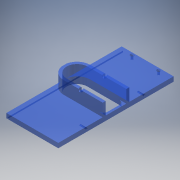
# Autodesk Inventor part: Wand1
Saved by Autodesk Inventor 2018 (Build 220112000, 112)
## iProperties
Created: 2013-02-21
Part Number: Wand1
Material: Polycarbonate, Smoke
Document SubType Name: Modeling
Designer: Neef
Mass: 105.37 g
Surface Area: 310.912 cm^2
Volume: 87.8083 cm^3
Density: 1.2 g/cm^3
Appearance: Clear - Blue
Author: Neef
Autodesk Inventor part; units mm, degrees
ref_plane "YZ Plane" through (0, 0, 0) normal (1, 0, 0) x (0, 1, 0)
ref_plane "XZ Plane" through (0, 0, 0) normal (0, 1, 0) x (-1, 0, 0)
ref_plane "XY Plane" through (0, 0, 0) normal (0, 0, 1) x (1, 0, 0)
sketch "Skizze1" plane through (0, 0, 0) normal (0, 0, 1) x (1, 0, 0)
  line L0 (45, 100) -> (-45, 100)
  line L1 (-45, 100) -> (-45, -100)
  line L2 (-45, -100) -> (45, -100)
  line L3 (45, -100) -> (45, 100)
  line L4 (0, 140) -> (0, -140) projected
  line L5 (-63, 0) -> (63, 0) projected
  point P0 (0, 0)
  point P1 (45, 0)
  point P2 (0, -100)
  dimension "d0" = 200
  dimension "d1" = 90
  constraints: 8 end point, 2 midpoint, 2 parallel, 2 point on line, 1 horizontal, 1 perpendicular
  measures "d0" distance of L2.end L0.start
  measures "d1" distance of L0.start L0.end
extrude "Extrusion1" add sketch "Skizze1" along normal blind 8
sketch "Skizze2" plane through (0, 0, 8) normal (0, 0, 1) x (1, 0, 0)
  line L0 (45, 100) -> (45, -100) projected
  line L1 (-45, -100) -> (-45, 100) projected
  line L2 (45, -18) -> (-22.5, -18)
  arc A0 (-40.5, 0) -> (-22.5, -18) centre (-22.5, 0) ccw
  line L3 (-40.5, 0) -> (-45, 0)
  arc A1 (-45, -4.7697) -> (-22.5, -23) centre (-22.5, 0) ccw
  line L4 (-22.5, -23) -> (45, -23)
  line L5 (0, 140) -> (0, -140) projected
  line L6 (-66.8751, 0) -> (63.6458, 0) projected
  line L7 (-45, -4.7697) -> (-45, 0)
  point P0 (0, 0)
  dimension "d4" = 5
  dimension "d5" = 67.5
  dimension "d6" = 18
  constraints: 8 end point, 5 point on line, 4 point on circle, 2 centre point, 2 perpendicular, 2 tangent, 1 collinear, 1 midpoint, 1 parallel
  measures "d4" distance between parallel lines of L2 L4
  measures "d5" distance of L2.start L2.end
  measures "d6" distance between parallel lines of L6 L2
extrude "Extrusion2" add sketch "Skizze2" along normal blind 22 contours L0 L4 L5 L2 | L5 L4 A1 L1 L3 A0 L2
mirror "Spiegeln1" about plane through (-45, 0, 8) normal (0, 1, 0) of "Extrusion2"
sketch "Skizze3" plane through (0, 0, 8) normal (0, 0, 1) x (1, 0, 0)
  line L0 (45, 18) -> (-22.5, 18) projected
  arc A0 (-22.5, 18) -> (-22.5, -18) centre (-22.5, 0) ccw projected
  line L1 (-22.5, -18) -> (45, -18) projected
  line L2 (45, 18) -> (45, -18) projected
  arc A1 (23, -18) -> (23, 18) centre (23, 0) ccw
  line L3 (-63, 0) -> (63, 0) projected
  line L4 (-22.5, 18) -> (45, 18) projected
  line L5 (-22.5, -18) -> (45, -18) projected
  point P0 (0, 0)
  dimension "d9" = 22
  constraints: 3 point on line, 2 point on circle, 2 tangent, 1 centre point
  measures "d9" distance from line of L2 A1.centre
extrude "Extrusion3" cut sketch "Skizze3" against normal through all contours A1 L3 A0 L0 | A1 L1 A0 L3
sketch "Skizze4" plane through (-45, 100, 0) normal (0, 1, 0) x (1, 0, 0)
  line L0 (90, 0) -> (0, 0) projected
  line L1 (0, 0) -> (0, -8) projected
  line L2 (22.5, -30) -> (22.5, -30) projected
  line L3 (22.5, -30) -> (22.5, 0) projected
  line L4 (22.5, 0) -> (22.5, 0) projected
  line L5 (22.5, 0) -> (22.5, -30) projected
  line L6 (4.5, -30) -> (4.5, 0) projected
  line L7 (2, 0) -> (3.2, 0)
  line L8 (3.2, 0) -> (3.2, -2.5)
  line L9 (3.2, -2.5) -> (2, -2.5)
  line L10 (2, -2.5) -> (2, 0)
  point P0 (45, 0)
  dimension "d12" = 1.2
  dimension "d13" = 2.5
  dimension "d14" = 2
  constraints: 8 end point, 2 parallel, 1 horizontal, 1 perpendicular, 1 point on line
  measures "d12" distance of L8.end L9.end
  measures "d13" distance of L9.end L7.start
  measures "d14" distance between parallel lines of L1 L10
extrude "Extrusion4" cut sketch "Skizze4" against normal through all
sketch "Skizze5" plane through (0, 0, 8) normal (0, 0, 1) x (1, 0, 0)
  arc A0 (23, -18) -> (23, 18) centre (23, 0) ccw projected
  line L0 (45, 18) -> (23, 18) projected
  line L1 (41, 0) -> (41, 10)
  line L2 (33, 18) -> (23, 18)
  arc A1 (41, 0) -> (23, 18) centre (23, 0) ccw
  arc A2 (41, 10) -> (33, 18) centre (33, 10) ccw
  point P0 (0, 0)
  point P1 (41, 18)
  dimension "d17" = 8
  constraints: 5 point on circle, 4 end point, 4 tangent, 3 point on line, 2 centre point, 1 coincident, 1 collinear, 1 perpendicular
  measures "d17" radius of A2
extrude "Extrusion5" cut sketch "Skizze5" against normal up to surface (8 mm away)
mirror "Spiegeln2" about plane through (0, 0, 0) normal (0, 1, 0) of "Extrusion5"
sketch "Skizze6" plane through (45, -100, 0) normal (1, 0, 0) x (0, 0, -1)
  line L0 (-8, 77) -> (-8, 0) projected
  line L1 (0, 0) -> (-8, 0) projected
  point P0 (0, 100)
  point P1 (-4, 50)
  dimension "d20" = 4
  dimension "d21" = 50
  measures "d20" distance from line of L0 point (-4, 50)
  measures "d21" distance from line of point (-4, 50) L1
hole "Bohrung1" at (45, -50, 4) direction (-1, 0, 0) diameter 2.459 depth 12 tip angle 118 thread size "M3x0.5" class "6H" standard "ISO Metric profile"
mirror "Spiegeln3" about plane through (0, 0, 0) normal (0, 1, 0) of "Bohrung1"
sketch "Skizze7" plane through (0, 0, 30) normal (0, 0, 1) x (1, 0, 0)
  line L0 (45, -18) -> (45, -23) projected
  line L1 (-22.5, 18) -> (45, 18) projected
  line L2 (45, 18) -> (45, 23) projected
  line L3 (45, -23) -> (-22.5, -23) projected
  point P0 (0, 0)
  point P1 (5, 20.5)
  point P2 (5, -20.5)
  dimension "d29" = 40
  dimension "d30" = 40
  dimension "d31" = 2.5
  dimension "d32" = 2.5
  measures "d29" distance from line of L2 point (5, 20.5)
  measures "d30" distance from line of point (5, -20.5) L0
  measures "d31" distance from line of point (5, -20.5) L3
  measures "d32" distance from line of L1 point (5, 20.5)
hole "Bohrung2" at (5, 20.5, 30) at (5, -20.5, 30) direction (0, 0, -1) diameter 5.6 depth 4
sketch "Skizze8" plane through (0, 0, 8) normal (0, 0, 1) x (1, 0, 0)
  line L0 (45, 100) -> (45, 23) projected
  line L1 (-45, 100) -> (45, 100) projected
  line L2 (-45, 4.7697) -> (-45, 100) projected
  point P0 (0, 0)
  point P1 (23, 96)
  point P2 (-23, 96)
  dimension "d40" = 22
  dimension "d41" = 22
  dimension "d42" = 4
  dimension "d43" = 4
  measures "d40" distance from line of L0 point (23, 96)
  measures "d41" distance from line of L2 point (-23, 96)
  measures "d42" distance from line of L1 point (23, 96)
  measures "d43" distance from line of L1 point (-23, 96)
hole "Bohrung3" at (23, 96, 8) at (-23, 96, 8) direction (0, 0, -1) diameter 3.4 end through all countersink diameter 6.3 countersink angle 90 clearance for "Flachkopfsenkschraube DIN EN ISO 2009" size "M3" standard "DIN"
equation "\"d30\" = d29"
equation "\"d41\" = d40"
equation "\"d43\" = d42"
